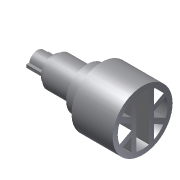
# Autodesk Inventor part: DrivingShaft
Saved by Autodesk Inventor 2012 (Build 160160000, 160)
## iProperties
Created: 2017-01-26
Part Number: DrivingShaft
Material: Default
Document SubType Name: Modeling
Designer: omaro
Density: 1 g/cm^3
Author: omaro
Autodesk Inventor part; units mm, degrees
ref_plane "YZ Plane" through (0, 0, 0) normal (1, 0, 0) x (0, 1, 0)
ref_plane "XZ Plane" through (0, 0, 0) normal (0, 1, 0) x (-1, 0, 0)
ref_plane "XY Plane" through (0, 0, 0) normal (0, 0, 1) x (1, 0, 0)
sketch "Sketch1" plane through (0, 0, 0) normal (0, 0, 1) x (1, 0, 0)
  line L0 (34.580292, 0) -> (34.580292, 11.9)
  line L1 (34.580292, 11.9) -> (28.380292, 11.9)
  line L2 (28.380292, 11.9) -> (18.180292, 11.9)
  line L3 (18.180292, 11.9) -> (18.180292, 8.45)
  line L4 (18.180292, 8.45) -> (12.580292, 8.45)
  line L5 (12.580292, 8.45) -> (12.580292, 6.05)
  line L6 (12.580292, 6.05) -> (0.680292, 6.05)
  line L7 (0.680292, 6.05) -> (0.680292, 5)
  line L8 (0.680292, 5) -> (-0.919708, 5)
  line L9 (-0.919708, 5) -> (-0.919708, 3.3)
  line L10 (-0.919708, 3.3) -> (-7.319708, 3.3)
  line L11 (-7.319708, 3.3) -> (-7.319708, 0)
  line L12 (-19.229424, 0) -> (45.657176, 0)
  line L13 (-7.319708, 0) -> (34.580292, 0)
  point P0 (0, 0)
  dimension "d0" = 11.9
  dimension "d1" = 6.2
  dimension "d2" = 10.2
  dimension "d3" = 3.45
  dimension "d4" = 5.6
  dimension "d5" = 2.4
  dimension "d6" = 11.9
  dimension "d7" = 1.05
  dimension "d8" = 1.6
  dimension "d9" = 1.7
  dimension "d54" = 6.4
  constraints: 28 end point, 6 perpendicular, 5 parallel, 2 collinear, 1 vertical
  measures "d0" distance of L0.start L0.end
  measures "d1" distance of L0.end L1.end
  measures "d2" distance of L1.end L2.end
  measures "d3" distance of L2.end L3.end
  measures "d4" distance of L3.end L4.end
  measures "d5" distance of L4.end L5.end
  measures "d6" distance of L5.end L6.end
  measures "d7" distance of L6.end L7.end
  measures "d8" distance of L7.end L8.end
  measures "d9" distance of L8.end L9.end
  measures "d54" distance between parallel lines of L9 L11
revolve "Revolution1" add sketch "Sketch1" angle 360 about axis through (-19.229424, 0, 0) along (1, 0, 0)
sketch "Sketch2" plane through (-7.319708, 0, 0) normal (-1, 0, 0) x (0, 0, 1)
  circle A0 centre (0, 0) radius 3.3 projected
  circle A1 centre (0, 0) radius 1.25
  dimension "d12" = 2.5
  constraints: 1 centre point, 1 coincident
  measures "d12" diameter of A1
extrude "Extrusion1" cut sketch "Sketch2" against normal through all contours A1
sketch "Sketch3" plane through (34.580292, 0, 0) normal (1, 0, 0) x (0, 0, -1)
  circle A0 centre (0, 0) radius 1.25
  circle A1 centre (0, 0) radius 11.9
  circle A2 centre (0, 0) radius 9.9
  line L0 (-9.579144, 2.5) -> (9.579144, 2.5)
  line L1 (1.244069, 4.49804) -> (3.713385, 9.177187)
  line L2 (3.506516, 4.5) -> (5.482105, 8.243575)
  line L3 (-0.869771, 4.49804) -> (-3.397213, 9.298868)
  line L4 (-3.130001, 4.49804) -> (-5.197777, 8.425741)
  line L5 (-8.819163, 4.49804) -> (-3.130001, 4.49804)
  line L6 (-0.869771, 4.49804) -> (1.244069, 4.49804)
  line L7 (3.506516, 4.5) -> (8.818163, 4.5)
  line L8 (-9.579144, -2.5) -> (9.579144, -2.5)
  line L9 (-3.397213, -4.5) -> (-5.400973, -8.296957)
  line L10 (-1.135801, -4.5) -> (-3.623092, -9.213208)
  line L11 (3.504299, -4.5) -> (5.476946, -8.247004)
  line L12 (1.244069, -4.5) -> (3.707642, -9.179509)
  line L13 (8.818163, -4.5) -> (3.504299, -4.5)
  line L14 (1.244069, -4.5) -> (-1.135801, -4.5)
  line L15 (-3.397213, -4.5) -> (-8.818163, -4.5)
  dimension "d16" = 19.8
  dimension "d15" = 23.8
  dimension "d18" = 2.5
  dimension "d19" = 2
  dimension "d20" = 2
  dimension "d24" = 2
  dimension "d25" = 2
  dimension "d26" = 2
  dimension "d28" = 2.5
  constraints: 32 end point, 13 parallel, 1 coincident, 1 horizontal, 18 other
  measures "d15" diameter of A1
  measures "d18" distance from line of A0.centre L0
  measures "d19" distance between parallel lines of L3 L4
  measures "d20" distance between parallel lines of L2 L1
  measures "d24" distance between parallel lines of L0 L7
  measures "d25" distance between parallel lines of L11 L12
  measures "d26" distance between parallel lines of L9 L10
  measures "d28" distance from line of A0.centre L8
extrude "Extrusion2" cut sketch "Sketch3" against normal blind 12 contours A2 L8 L0 | L7 L2 A2 | A2 L11 L13 | A2 L4 L5 | L15 L9 A2 | L1 L6 L3 A2 | A2 L10 L14 L12
sketch "Sketch4" plane through (-7.319708, 0, 0) normal (-1, 0, 0) x (0, 0, 1)
  circle A0 centre (0, 0) radius 1.25
  circle A1 centre (0, 0) radius 3.3
  line L0 (-0.602013, 3.244623) -> (-0.602013, 4.4)
  line L1 (0, 7.165541) -> (0, -7.239273)
  arc A2 (-0.602013, -3.258413) -> (0.597987, -3.239718) centre (-0.052561, -0.004477) ccw
  arc A3 (0.597987, 3.2259) -> (-0.602013, 3.244623) centre (-0.052561, -0.004477) ccw
  line L2 (-7.277237, 0) -> (-5, 0)
  line L3 (-3.3, 0) -> (3.3, 0)
  line L4 (5, 0) -> (7.340981, 0)
  line L5 (0.597987, 4.4) -> (0.597987, 3.2259)
  line L6 (-0.602013, 4.4) -> (0.597987, 4.4)
  line L7 (-0.602013, -4.4) -> (0.597987, -4.4)
  line L8 (-0.602013, -4.4) -> (-0.602013, -3.244623)
  line L9 (0.597987, -4.4) -> (0.597987, -3.239718)
  dimension "d32" = 0
  dimension "d40" = 4.4
  dimension "d42" = 1.2
  dimension "d44" = 1.2
  constraints: 20 end point, 6 perpendicular, 6 point on circle, 2 centre point, 2 parallel, 2 symmetric about line, 1 point on line, 1 vertical
  measures "d32" distance from line of A0.centre L1
  measures "d40" distance from line of A0.centre L6
  measures "d42" distance between parallel lines of L5 L0
  measures "d44" distance between parallel lines of L9 L8
sketch "Sketch4 outline for Extrusion3" plane through (-7.319708, 0, 0) normal (-1, 0, 0) x (0, 0, 1)
  line L0 (-0.602013, -3.258413) -> (-0.602013, -4.4)
  arc A0 (0.597987, -3.239718) -> (-0.602013, -3.258413) centre (-0.052561, -0.004477) cw
  line L1 (0.597987, -4.4) -> (0.597987, -3.239718)
  line L2 (-0.602013, -4.4) -> (0.597987, -4.4)
  line L3 (-0.602013, 4.4) -> (-0.602013, 3.244623)
  line L4 (0.597987, 4.4) -> (-0.602013, 4.4)
  line L5 (0.597987, 3.2259) -> (0.597987, 4.4)
  arc A1 (-0.602013, 3.244623) -> (0.597987, 3.2259) centre (-0.052561, -0.004477) cw
extrude "Extrusion3" add sketch "Sketch4 outline for Extrusion3" against normal blind 7
sketch "Sketch5" plane through (22.580292, 0, 0) normal (1, 0, 0) x (0, 0, -1)
  circle A0 centre (0, 0) radius 1.25
  line L0 (9.579144, 2.5) -> (-9.579144, 2.5)
  arc A1 (-9.579144, 2.5) -> (-9.579144, -2.5) centre (0, 0) ccw
  circle A2 centre (0, 0) radius 2.5
  constraints: 1 centre point, 1 coincident, 1 tangent
extrude "Extrusion4" cut sketch "Sketch5" against normal blind 23
sketch "Sketch7" plane through (34.580292, 0, 0) normal (1, 0, 0) x (0, 0, -1)
  line L0 (9.579144, -2.5) -> (-9.579144, -2.5)
  line L1 (-9.579144, 2.5) -> (9.579144, 2.5)
  circle A0 centre (0, 0) radius 11.9
  arc A1 (7.071068, -2.5) -> (7.071068, 2.5) centre (0, 0) ccw
  arc A2 (-7.071068, 2.5) -> (-7.071068, -2.5) centre (0, 0) ccw
  dimension "d49" = 7.5
  dimension "d50" = 7.5
  constraints: 4 point on circle, 4 point on line, 2 centre point, 1 coincident
  measures "d49" radius of A1
  measures "d50" radius of A2
extrude "Extrusion5" cut sketch "Sketch7" against normal blind 14 contours L0 A2 L1 A1
sketch "Sketch8" plane through (34.580292, 0, 0) normal (1, 0, 0) x (0, 0, -1)
  line L0 (9.579144, -2.5) -> (-9.579144, -2.5)
  line L1 (-9.579144, 2.5) -> (9.579144, 2.5)
  arc A0 (-7.071068, 2.5) -> (-7.071068, -2.5) centre (0, 0) ccw
  arc A1 (7.071068, -2.5) -> (7.071068, 2.5) centre (0, 0) ccw
  arc A2 (6.538348, -2.5) -> (6.538348, 2.5) centre (0, 0) ccw
  arc A3 (-6.538348, 2.5) -> (-6.538348, -2.5) centre (0, 0) ccw
  constraints: 4 point on circle, 4 point on line, 2 centre point, 1 coincident
extrude "Extrusion6" cut sketch "Sketch8" against normal blind 20 contours L0 A3 L1 A2
equation "\"d50\" = d49"
body "Solid1"
